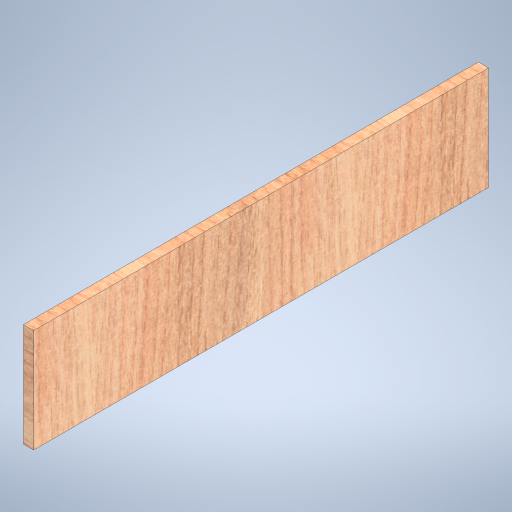
# Autodesk Inventor part: Grundfläche
Saved by Autodesk Inventor 2023 (Build 270158000, 158)
## iProperties
Created: 2024-01-25
Part Number: Grundfläche
Material: Generisch
Document SubType Name: Modeling
Designer: phili
Density: 1 g/cm^3
Appearance: Vorgabe
Author: phili
Autodesk Inventor part; units mm, degrees
ref_plane "YZ Plane" through (0, 0, 0) normal (1, 0, 0) x (0, 1, 0)
ref_plane "XZ Plane" through (0, 0, 0) normal (0, 1, 0) x (-1, 0, 0)
ref_plane "XY Plane" through (0, 0, 0) normal (0, 0, 1) x (1, 0, 0)
sketch "Skizze1" plane through (0, 0, 0) normal (1, 0, 0) x (0, 1, 0)
  line L0 (-50, -220) -> (50, -220)
  line L1 (50, -220) -> (50, 220)
  line L2 (50, 220) -> (-50, 220)
  line L3 (-50, 220) -> (-50, -220)
  line L4 (-50, -220) -> (50, 220) construction
  line L5 (50, -220) -> (-50, 220) construction
  point P0 (0, 0)
  dimension "d0" = 100
  dimension "d1" = 440
  constraints: 12 end point, 2 midpoint, 2 parallel, 1 horizontal, 1 perpendicular
  measures "d0" distance of L2.end L1.end
  measures "d1" distance of L1.end L0.end
extrude "Extrusion1" add sketch "Skizze1" along normal blind 10
